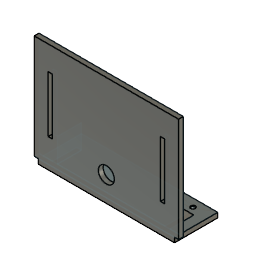
tcrt-adapter (Autodesk Fusion 360 design; units mm, degrees)
part number: 2026-06-21-19-30-25-528
part number: 2026-06-21-19-41-13-210
part number: 2026-06-21-22-05-45-043
Autodesk Fusion 360 part; units mm, degrees
sketch "Sketch1" plane through (0, 0, 0) normal (0, 0, 1) x (1, 0, 0) in component "TCRT_Chassis_Adapter"
  line L0 (-45, 12.5) -> (45, 12.5)
  line L1 (45, 12.5) -> (45, -12.5)
  line L2 (45, -12.5) -> (-45, -12.5)
  line L3 (-45, -12.5) -> (-45, 12.5)
  line L4 (-45, 12.5) -> (45, -12.5) construction
  line L5 (45, 12.5) -> (-45, -12.5) construction
  dimension "d18" = 90
  dimension "d19" = 25
  constraint horizontal L0
  constraint perpendicular L0 L1
  constraint parallel L0 L2
  constraint parallel L1 L3
  constraint coincident L4 origin
  constraint coincident L5 origin
  measures "d18" distance of L0.start L0.end
  measures "d19" distance of L0.start L2.end
extrude "Extrude1" add sketch "Sketch1" along normal blind 3 makes body 1 in component "TCRT_Chassis_Adapter"
sketch "Sketch2" plane through (0, 0, 3) normal (0, 0, 1) x (-1, 0, 0) in component "TCRT_Chassis_Adapter"
  line L0 (45, 12.5) -> (-45, 12.5)
  line L1 (-45, 12.5) -> (-45, -12.5)
  line L2 (-45, -12.5) -> (45, -12.5)
  line L3 (45, -12.5) -> (45, 12.5)
  line L4 (21, 1.3) -> (39, 1.3)
  line L5 (39, 1.3) -> (39, -1.3)
  line L6 (39, -1.3) -> (21, -1.3)
  line L7 (21, -1.3) -> (21, 1.3)
  line L8 (21, 1.3) -> (39, -1.3) construction
  line L9 (39, 1.3) -> (21, -1.3) construction
  line L10 (0, -12.5) -> (0, 12.5)
  line L11 (-39, -1.3) -> (-21, -1.3)
  line L12 (-39, 1.3) -> (-21, -1.3) construction
  line L13 (-21, -1.3) -> (-21, 1.3)
  line L14 (-21, 1.3) -> (-39, -1.3) construction
  line L15 (-21, 1.3) -> (-39, 1.3)
  line L16 (-39, 1.3) -> (-39, -1.3)
  point P0 (30, 0)
  point P1 (-30, 0)
  dimension "d22" = 18
  dimension "d23" = 30
  dimension "d24" = 2.6
  constraint horizontal L4
  constraint perpendicular L4 L5
  constraint parallel L4 L6
  constraint parallel L5 L7
  constraint coincident L8 P0
  constraint coincident L9 P0
  constraint midpoint L2 L10.start
  constraint midpoint L0 L10.end
  constraint symmetric L4.start L10 L13.end
  constraint symmetric L4.end L10 L12.start
  constraint symmetric L5.end L10 L11.start
  constraint symmetric L6.end L10 L11.end
  constraint symmetric P0 L10 P1
  measures "d22" distance of L5.end L6.end
  measures "d23" horizontal distance of origin P0
  measures "d24" distance of L4.end L5.end
extrude "Extrude2" cut sketch "Sketch2" against normal blind 8 contours L4 L5 L6 L7 | L11 L13 L15 L16 bodies 1 in component "TCRT_Chassis_Adapter"
sketch "Sketch3" plane through (0, 12.5, 0) normal (0, 1, 0) x (-1, 0, 0) in component "TCRT_Chassis_Adapter"
  line L0 (-45, 0) -> (45, 0)
  line L1 (45, 0) -> (45, 3)
  line L2 (45, 3) -> (-45, 3)
  line L3 (-45, 3) -> (-45, 0)
  line L4 (-45, 0) -> (45, 0)
  line L5 (45, 0) -> (45, -25)
  line L6 (45, -25) -> (-45, -25)
  line L7 (-45, -25) -> (-45, 0)
  constraint perpendicular L4 L5
  constraint parallel L4 L6
  constraint parallel L5 L7
  constraint coincident L0.end L1.start
  constraint perpendicular L1 L4
  constraint coincident L0.start L3.end
extrude "Extrude3" add sketch "Sketch3" against normal blind 4 contours L0 L4 L5 L6 L7 bodies 1 in component "TCRT_Chassis_Adapter"
sketch "Sketch4" plane through (0, 12.5, 0) normal (0, 1, 0) x (-1, 0, 0) in component "TCRT_Chassis_Adapter"
  line L0 (45, -25) -> (45, 3)
  line L1 (45, 3) -> (-45, 3)
  line L2 (-45, 3) -> (-45, -25)
  line L3 (-45, -25) -> (45, -25)
  circle A0 centre (-35, -12.5) radius 1.15
  line L4 (-0.2279, 3) -> (0, -25)
  circle A1 centre (34.7919, -11.932) radius 1.15
  dimension "d29" = 2.3
  dimension "d31" = 15.5
  constraint coincident L1 L4.start
  constraint midpoint L3 L4.end
  constraint symmetric A0 L4 A1
  measures "d29" diameter of A0
  measures "d31" distance of L1 A0.centre
sketch "Sketch1 (2)" plane through (0, 0, 0) normal (0, 1, 0) x (1, 0, 0) in component "TCRT_Sensor_Slider"
  line L0 (45, 32.5) -> (-45, 32.5)
  line L1 (-45, 32.5) -> (-45, -32.5)
  line L2 (-45, -32.5) -> (45, -32.5)
  line L3 (45, -32.5) -> (45, 32.5)
  line L4 (45, 32.5) -> (-45, -32.5) construction
  line L5 (-45, 32.5) -> (45, -32.5) construction
  dimension "d41" = 65
  dimension "d42" = 90
  constraint horizontal L0
  constraint perpendicular L0 L1
  constraint parallel L0 L2
  constraint parallel L1 L3
  constraint coincident L4 origin
  constraint coincident L5 origin
  measures "d41" distance of L0.start L2.end
  measures "d42" distance of L0.start L0.end
extrude "Extrude1'" add sketch "Sketch1 (2)" along normal blind 3 separate body makes body 2 in component "TCRT_Sensor_Slider"
sketch "Sketch2 (2)" plane through (0, 0, 0) normal (0, -1, 0) x (1, 0, 0) in component "TCRT_Sensor_Slider"
  line L0 (45, -32.5) -> (45, 32.5)
  line L1 (45, 32.5) -> (-45, 32.5)
  line L2 (-45, 32.5) -> (-45, -32.5)
  line L3 (-45, -32.5) -> (45, -32.5)
  line L4 (0, 32.5) -> (0, -32.5)
  line L5 (-33.7, -17.5001) -> (-36.3, -17.5001)
  line L6 (-36.3, -17.5001) -> (-36.3, 17.4999)
  line L7 (-36.3, 17.4999) -> (-33.7, 17.4999)
  line L8 (-33.7, 17.4999) -> (-33.7, -17.5001)
  line L9 (-33.7, -17.5001) -> (-36.3, 17.4999) construction
  line L10 (-36.3, -17.5001) -> (-33.7, 17.4999) construction
  line L11 (36.3, -17.5001) -> (33.7, 17.4999) construction
  line L12 (33.7, 17.4999) -> (33.7, -17.5001)
  line L13 (33.7, -17.5001) -> (36.3, -17.5001)
  line L14 (36.3, 17.4999) -> (33.7, 17.4999)
  line L15 (33.7, -17.5001) -> (36.3, 17.4999) construction
  line L16 (36.3, -17.5001) -> (36.3, 17.4999)
  point P0 (-35, -0.0001)
  point P1 (35, -0.0001)
  dimension "d45" = 35
  dimension "d46" = 2.6
  dimension "d47" = 35
  constraint midpoint L1 L4.start
  constraint midpoint L3 L4.end
  constraint horizontal L5
  constraint perpendicular L5 L6
  constraint parallel L5 L7
  constraint parallel L6 L8
  constraint coincident L9 P0
  constraint coincident L10 P0
  constraint symmetric L4 L5.start L12.end
  constraint symmetric L4 L5.end L11.start
  constraint symmetric L4 L6.end L14.start
  constraint symmetric L4 L7.end L11.end
  constraint symmetric L4 P0 P1
  measures "d45" distance of L5.end L6.end
  measures "d46" distance of L6.end L7.end
  measures "d47" distance of L4 P0
extrude "Extrude2'" cut sketch "Sketch2 (2)" against normal blind 3 contours L5 L6 L7 L8 | L12 L13 L14 L16 bodies 2 in component "TCRT_Sensor_Slider"
sketch "Sketch3 (2)" plane through (0, 0, 0) normal (1, 0, 0) x (0, 1, 0) in component "TCRT_Sensor_Slider"
sketch "Sketch4 (2)" plane through (0, 0, -32.5) normal (0, 0, -1) x (1, 0, 0) in component "TCRT_Sensor_Slider"
  line L0 (45, 0) -> (-45, 0)
  line L1 (-45, 0) -> (-45, -3)
  line L2 (-45, -3) -> (45, -3)
  line L3 (45, -3) -> (45, 0)
sketch "Sketch5" plane through (0, 0, -32.5) normal (0, 0, -1) x (1, 0, 0) in component "TCRT_Sensor_Slider"
  line L0 (-42.5, 0) -> (42.5, 0)
  line L1 (42.5, 0) -> (42.5, -27)
  line L2 (42.5, -27) -> (-42.5, -27)
  line L3 (-42.5, -27) -> (-42.5, 0)
  dimension "d50" = 42.5
  dimension "d51" = 42.5
  dimension "d52" = 27
  constraint perpendicular L0 L1
  constraint parallel L0 L2
  constraint parallel L1 L3
  constraint horizontal L0
  measures "d50" distance of L0.start origin
  measures "d51" distance of L0.end origin
  measures "d52" distance of L0.end L1.end
extrude "Extrude3'" add sketch "Sketch5" along normal blind 3 bodies 2 in component "TCRT_Sensor_Slider"
sketch "Sketch6" plane through (0, 3, 0) normal (0, 1, 0) x (-1, 0, 0) in component "TCRT_Sensor_Slider"
  line L0 (36.3, 17.4999) -> (36.3, -17.5001)
  line L1 (36.3, -17.5001) -> (33.7, -17.5001)
  line L2 (33.7, -17.5001) -> (33.7, 17.4999)
  line L3 (33.7, 17.4999) -> (36.3, 17.4999)
  line L4 (-36.3, 17.4999) -> (-33.7, 17.4999)
  line L5 (-33.7, 17.4999) -> (-33.7, -17.5001)
  line L6 (-33.7, -17.5001) -> (-36.3, -17.5001)
  line L7 (-36.3, -17.5001) -> (-36.3, 17.4999)
  line L8 (-45, 32.5) -> (-45, -32.5)
  line L9 (-45, -32.5) -> (-42.5, -32.5)
  line L10 (-42.5, -32.5) -> (42.5, -32.5)
  line L11 (42.5, -32.5) -> (45, -32.5)
  line L12 (45, -32.5) -> (45, 32.5)
  line L13 (45, 32.5) -> (-45, 32.5)
sketch "Sketch7" plane through (0, 3, 0) normal (0, 1, 0) x (-1, 0, 0) in component "TCRT_Sensor_Slider"
  line L0 (-33.5, -32.5) -> (-36.5, -32.5)
  line L1 (-36.5, -32.5) -> (-36.5, -17.5)
  line L2 (-36.5, -17.5) -> (-33.5, -17.5)
  line L3 (-33.5, -17.5) -> (-33.5, -32.5)
  line L4 (-33.5, -32.5) -> (-36.5, -17.5) construction
  line L5 (-36.5, -32.5) -> (-33.5, -17.5) construction
  line L6 (0, 32.5) -> (0, -32.5)
  line L7 (36.5, -17.5) -> (33.5, -17.5)
  line L8 (36.5, -32.5) -> (33.5, -17.5) construction
  line L9 (36.5, -32.5) -> (36.5, -17.5)
  line L10 (33.5, -32.5) -> (36.5, -17.5) construction
  line L11 (33.5, -17.5) -> (33.5, -32.5)
  line L12 (33.5, -32.5) -> (36.5, -32.5)
  point P0 (-35, -25)
  dimension "d57" = 3
  dimension "d58" = 15
  constraint horizontal L0
  constraint perpendicular L0 L1
  constraint parallel L0 L2
  constraint parallel L1 L3
  constraint coincident L4 P0
  constraint coincident L5 P0
  constraint symmetric L0.start L6 L10.start
  constraint symmetric L0.end L6 L8.start
  constraint symmetric L1.end L6 L7.start
  constraint symmetric L2.end L6 L7.end
  measures "d57" distance of L1.end L2.end
  measures "d58" distance of L0.end L1.end
extrude "Extrude4" add sketch "Sketch7" along normal blind 15 bodies 2 in component "TCRT_Sensor_Slider"
sketch "Sketch8" plane through (36.5, 0, 0) normal (1, 0, 0) x (0, 1, 0) in component "TCRT_Sensor_Slider"
  line L0 (3, -17.5) -> (3, -32.5)
  line L1 (3, -32.5) -> (18, -32.5)
  line L2 (18, -32.5) -> (18, -17.5)
  line L3 (18, -17.5) -> (3, -17.5)
  line L4 (3, -17.5) -> (18, -32.5)
  line L5 (3, -17.5) -> (18, -17.5)
  line L6 (18, -32.5) -> (18, -17.5)
  constraint coincident L0.start L3.end
  constraint coincident L1.end L2.start
  constraint coincident L2.end L3.start
extrude "Extrude5" cut sketch "Sketch8" against normal blind 3 contours L2 L3 L4 L5 L6 bodies 2 in component "TCRT_Sensor_Slider"
sketch "Sketch9" plane through (-33.5, 0, 0) normal (1, 0, 0) x (0, 1, 0) in component "TCRT_Sensor_Slider"
  line L0 (3, -17.5) -> (3, -32.5)
  line L1 (3, -32.5) -> (18, -32.5)
  line L2 (18, -32.5) -> (18, -17.5)
  line L3 (18, -17.5) -> (3, -17.5)
sketch "Sketch10" plane through (-36.5, 0, 0) normal (-1, 0, 0) x (0, -1, 0) in component "TCRT_Sensor_Slider"
  line L0 (-3, -32.5) -> (-3, -17.5)
  line L1 (-3, -17.5) -> (-18, -17.5)
  line L2 (-18, -17.5) -> (-18, -32.5)
  line L3 (-18, -32.5) -> (-3, -32.5)
  line L4 (-18, -32.5) -> (-3, -17.5)
  line L5 (-3, -17.5) -> (-18, -17.5)
  line L6 (-18, -32.5) -> (-18, -17.5)
  constraint coincident L2.end L3.start
  constraint coincident L0.end L1.start
  constraint coincident L1.end L2.start
extrude "Extrude6" cut sketch "Sketch10" against normal blind 3 contours L1 L2 L4 L5 L6 bodies 2 in component "TCRT_Sensor_Slider"
extrude "Extrude5'" cut sketch "Sketch4" against normal blind 5 contours A0 bodies 1 in component "TCRT_Chassis_Adapter"
extrude "Extrude6'" cut sketch "Sketch4" against normal blind 5 contours A1 bodies 1 in component "TCRT_Chassis_Adapter"
fillet "Fillet2" radius 0.3 2 edges at (36.0722, 12.5, -12.0841) (-33.7197, 12.5, -11.5161) on bodies 1 in component "TCRT_Chassis_Adapter"
sketch "Sketch11" plane through (0, 0, -32.5) normal (0, 0, 1) x (-1, 0, 0) in component "TCRT_Sensor_Slider"
  line L0 (33.5, -18) -> (33.5, -3)
  line L1 (33.5, -3) -> (-33.5, -3)
  line L2 (-33.5, -3) -> (-33.5, -18)
  line L3 (-33.5, -18) -> (-36.5, -18)
  line L4 (-36.5, -18) -> (-36.5, -3)
  line L5 (-36.5, -3) -> (-42.5, -3)
  line L6 (-42.5, -3) -> (-42.5, -27)
  line L7 (-42.5, -27) -> (42.5, -27)
  line L8 (42.5, -27) -> (42.5, -3)
  line L9 (42.5, -3) -> (36.5, -3)
  line L10 (36.5, -3) -> (36.5, -18)
  line L11 (36.5, -18) -> (33.5, -18)
sketch "Sketch12" plane through (0, 0, -32.5) normal (0, 0, 1) x (-1, 0, 0) in component "TCRT_Sensor_Slider"
  circle A0 centre (0, -22) radius 1.15
  circle A1 centre (-16, -22) radius 1.15
  circle A2 centre (-32, -22) radius 1.15
  circle A3 centre (32, -22) radius 1.15
  circle A4 centre (16, -22) radius 1.15
  dimension "d71" = 2.3
  dimension "d72" = 2.3
  dimension "d73" = 16
  dimension "d74" = 2.3
  dimension "d75" = 16
  measures "d71" diameter of A0
  measures "d72" diameter of A1
  measures "d73" distance of A0.centre A1.centre
  measures "d74" diameter of A2
  measures "d75" distance of A1.centre A2.centre
extrude "Extrude7" cut sketch "Sketch12" against normal blind 5 bodies 2 in component "TCRT_Sensor_Slider"
sketch "Sketch13" plane through (0, 3, 0) normal (0, 1, 0) x (-1, 0, 0) in component "TCRT_Sensor_Slider"
  circle A0 centre (0, -20) radius 5
  dimension "d78" = 10
  measures "d78" diameter of A0
extrude "Extrude8" cut sketch "Sketch13" against normal blind 15 bodies 2 in component "TCRT_Sensor_Slider"
chamfer "Chamfer1" distance 0.3 angle 45 1 edges at (33.0722, 21.5841, -32.5) on bodies 2 in component "TCRT_Sensor_Slider"
chamfer "Chamfer2" distance 0.3 angle 45 1 edges at (17.0722, 21.5841, -32.5) on bodies 2 in component "TCRT_Sensor_Slider"
chamfer "Chamfer3" distance 0.3 angle 45 1 edges at (1.0722, 21.5841, -32.5) on bodies 2 in component "TCRT_Sensor_Slider"
chamfer "Chamfer4" distance 0.3 angle 45 1 edges at (-14.9278, 21.5841, -32.5) on bodies 2 in component "TCRT_Sensor_Slider"
chamfer "Chamfer5" distance 0.3 angle 45 1 edges at (-30.9278, 21.5841, -32.5) on bodies 2 in component "TCRT_Sensor_Slider"
component "TCRT_Chassis_Adapter" placed x (1, 0, 0) y (0, 1, 0) z (0, 0, 1) at (0, 0, 0)
component "TCRT_Sensor_Slider" placed x (1, 0, 0) y (0, 1, 0) z (0, 0, 1) at (0, 0, 0)
equation "adapter_width = 90 mm"
equation "adapter_depth = 25 mm"
equation "plate_thickness = 3 mm"
equation "front_wall_height = 25 mm"
equation "front_wall_thickness = 4 mm"
equation "slider_width = 90 mm"
equation "slider_height = 65 mm"
equation "slider_thickness = 3 mm"
equation "sensor_shelf_width = 85 mm"
equation "sensor_shelf_depth = 24 mm"
equation "sensor_shelf_thickness = 3 mm"
equation "vertical_slot_height = 35"
equation "slot_width = 4.2 mm"
equation "sensor_spacing = 13 mm"
equation "zip_slot_width = 3.5 mm"
equation "zip_slot_length = 10 mm"
equation "m3_clearance = 3.2 mm"
